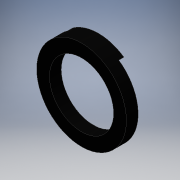
# Autodesk Inventor part: Toggle_Collar
Saved by Autodesk Inventor 2016 (Build 200138000, 138)
## iProperties
Created: 2016-04-13
Part Number: Toggle_Collar
Material: PC/ABS Plastic
Document SubType Name: Modeling
Designer: agmle
Density: 0.357273 g/cm^3
Appearance: Smooth - Black
Author: agmle
Autodesk Inventor part; units mm, degrees
ref_plane "YZ Plane" through (0, 0, 0) normal (1, 0, 0) x (0, 1, 0)
ref_plane "XZ Plane" through (0, 0, 0) normal (0, 1, 0) x (-1, 0, 0)
ref_plane "XY Plane" through (0, 0, 0) normal (0, 0, 1) x (1, 0, 0)
sketch "Sketch1" plane through (0, 0, 0) normal (0, 1, 0) x (-1, 0, 0)
  circle A0 centre (0, 0) radius 8.75
  circle A1 centre (0, 0) radius 6.25
  dimension "d0" = 17.5
  dimension "d1" = 12.5
  constraints: 2 centre point, 2 coincident
  measures "d0" diameter of A0
  measures "d1" diameter of A1
extrude "Extrusion1" add sketch "Sketch1" along normal blind 3.3
sketch "Sketch2" plane through (0, 3.3, 0) normal (0, 1, 0) x (1, 0, 0)
  circle A0 centre (0, 0) radius 8.75 projected
  line L0 (-4.9722, -7.2) -> (4.9722, -7.2)
  line L1 (4.9722, 7.2) -> (-4.9722, 7.2)
  line L2 (-12.7989, 0) -> (12.7989, 0) construction
  dimension "d4" = 14.4
  constraints: 6 end point, 4 point on circle, 1 coincident, 1 horizontal, 1 midpoint, 1 parallel
  measures "d4" distance between parallel lines of L1 L0
extrude "Extrusion2" cut sketch "Sketch2" against normal blind 1 contours A0 L0 L1
body "Solid1"
